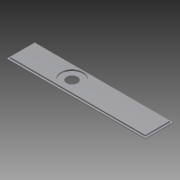
# Autodesk Inventor part: Tapa
Saved by Autodesk Inventor 2011 (Build 150239000, 239)
## iProperties
Created: 2014-08-05
Part Number: Tapa
Document SubType Name: Modeling
Designer: Admin
Density: 1 g/cm^3
Author: Admin
Autodesk Inventor part; units mm, degrees
ref_plane "YZ Plane" through (0, 0, 0) normal (1, 0, 0) x (0, 1, 0)
ref_plane "XZ Plane" through (0, 0, 0) normal (0, 1, 0) x (-1, 0, 0)
ref_plane "XY Plane" through (0, 0, 0) normal (0, 0, 1) x (1, 0, 0)
sketch "Boceto1" plane through (0, 0, 0) normal (0, 0, 1) x (1, 0, 0)
  line L0 (0, 0) -> (200, 0)
  line L1 (200, 0) -> (200, 40)
  line L2 (200, 40) -> (0, 40)
  line L3 (0, 40) -> (0, 0)
  circle A0 centre (74, 20) radius 8
  dimension "d0" = 200
  dimension "d1" = 40
  dimension "d2" = 16
  dimension "d3" = 74
  dimension "d4" = 20
  constraints: 8 end point, 2 parallel, 1 centre point, 1 horizontal, 1 perpendicular
  measures "d0" distance of L2.end L1.end
  measures "d1" distance of L1.end L0.end
  measures "d2" diameter of A0
  measures "d3" distance from line of L3 A0.centre
  measures "d4" distance from line of L0 A0.centre
extrude "Extrusión1" add sketch "Boceto1" along normal blind 1
sketch "Boceto2" plane through (0, 0, 1) normal (0, 0, 1) x (1, 0, 0)
  circle A0 centre (74, 20) radius 8 projected
  line L0 (0, 0) -> (0, 40) projected
  line L1 (200, 0) -> (0, 0) projected
  line L2 (200, 40) -> (200, 0) projected
  line L3 (0, 40) -> (200, 40) projected
  line L4 (197.9, 37.9) -> (197.9, 2.1)
  line L5 (197.9, 2.1) -> (2.1, 2.1)
  line L6 (2.1, 2.1) -> (2.1, 37.9)
  line L7 (2.1, 37.9) -> (197.9, 37.9)
  circle A1 centre (74, 20) radius 16
  dimension "d7" = 2.1
  dimension "d8" = 32
  constraints: 8 end point, 1 centre point, 1 concentric, 3 other
  measures "d7" horizontal distance of L6.end L0.end
  measures "d8" diameter of A1
extrude "Extrusión2" add sketch "Boceto2" along normal blind 2 contours L4 L5 L6 L7
